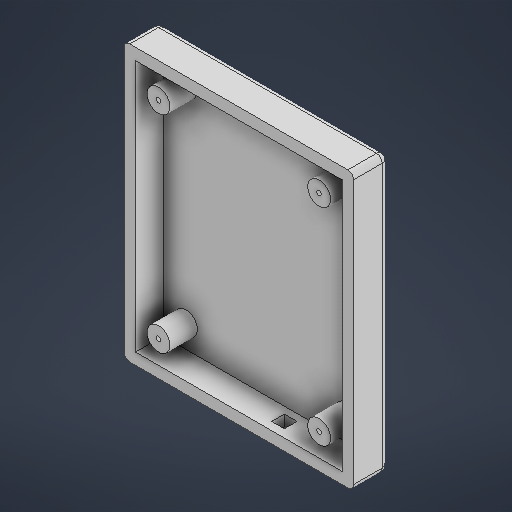
# Autodesk Inventor part: Bottom_Shell
Saved by Autodesk Inventor 2026.2 (Build 302298010, 298A)
## iProperties
Created: 2026-03-03
Part Number: Bottom_Shell
Material: Generic
Document SubType Name: Modeling
Designer: kjedr
Density: 1 g/cm^3
Appearance: Default
Author: kjedr
Autodesk Inventor part; units mm, degrees
ref_plane "YZ Plane" through (0, 0, 0) normal (1, 0, 0) x (0, 1, 0)
ref_plane "XZ Plane" through (0, 0, 0) normal (0, 1, 0) x (-1, 0, 0)
ref_plane "XY Plane" through (0, 0, 0) normal (0, 0, 1) x (1, 0, 0)
sketch "Sketch1" plane through (0, 0, 0) normal (0, 0, 1) x (1, 0, 0)
  line L0 (0, 0) -> (127, 0)
  line L1 (127, 0) -> (127, 152.4)
  line L2 (127, 152.4) -> (0, 152.4)
  line L3 (0, 152.4) -> (0, 0)
  dimension "d0" = 127
  dimension "d1" = 152.4
  constraints: 8 end point, 2 parallel, 1 horizontal, 1 perpendicular
  measures "d0" distance of L2.end L1.end
  measures "d1" distance of L1.end L0.end
extrude "Extrusion1" add sketch "Sketch1" along normal blind 19.05
sketch "Sketch2" plane through (0, 0, 19.05) normal (0, 0, 1) x (1, 0, 0)
  line L0 (6.35, 6.35) -> (120.65, 6.35)
  line L1 (120.65, 6.35) -> (120.65, 146.05)
  line L2 (120.65, 146.05) -> (6.35, 146.05)
  line L3 (6.35, 146.05) -> (6.35, 6.35)
  line L4 (0, 152.4) -> (0, 0) projected
  line L5 (0, 0) -> (127, 0) projected
  line L6 (127, 0) -> (127, 152.4) projected
  line L7 (127, 152.4) -> (0, 152.4) projected
  point P0 (127, 76.2)
  dimension "d4" = 6.35
  dimension "d5" = 6.35
  dimension "d6" = 6.35
  dimension "d7" = 6.35
  constraints: 8 end point, 2 parallel, 1 horizontal, 1 midpoint, 1 perpendicular
  measures "d4" distance between parallel lines of L4 L3
  measures "d5" distance between parallel lines of L5 L0
  measures "d6" distance from line of point (127, 76.2) L1
  measures "d7" distance between parallel lines of L7 L2
extrude "Extrusion2" cut sketch "Sketch2" against normal blind 15.24 contours L3 L2 L1 L0
fillet "Fillet1" radius 3.175 8 edges at (63.5, 152.4, 0) (127, 76.2, 0) (127, 0, 9.525) (0, 76.2, 0) (63.5, 0, 0) (127, 152.4, 9.525) (0, 152.4, 9.525) (0, 0, 9.525)
sketch "Sketch5" plane through (0, 0, 3.81) normal (0, 0, 1) x (1, 0, 0)
  circle A0 centre (19.05, 133.35) radius 6.35
  circle A1 centre (107.95, 133.35) radius 6.35
  circle A2 centre (19.05, 19.05) radius 6.35
  circle A3 centre (107.95, 19.05) radius 6.35
  line L0 (6.35, 6.35) -> (6.35, 146.05) projected
  line L1 (6.35, 146.05) -> (120.65, 146.05) projected
  line L2 (120.65, 146.05) -> (120.65, 6.35) projected
  line L3 (120.65, 6.35) -> (6.35, 6.35) projected
  point P0 (0, 0)
  dimension "d11" = 12.7
  dimension "d12" = 12.7
  dimension "d13" = 12.7
  dimension "d14" = 12.7
  dimension "d15" = 12.7
  constraints: 4 centre point, 3 equal radius, 2 horizontal alignment, 2 vertical alignment
  measures "d11" diameter of A0
  measures "d12" distance from line of L0 A0.centre
  measures "d13" distance from line of L1 A0.centre
  measures "d14" distance from line of L2 A1.centre
  measures "d15" distance from line of L3 A3.centre
extrude "Extrusion3" add sketch "Sketch5" along normal blind 15.24 contours A0 | A1 | A2 | A3
sketch "Sketch6" plane through (0, 0, 3.81) normal (0, 0, 1) x (1, 0, 0)
  line L0 (28.231, 93.35) -> (98.769, 93.35) construction
  line L1 (98.769, 93.35) -> (98.769, 9.35) construction
  line L2 (98.769, 9.35) -> (28.231, 9.35) construction
  line L3 (28.231, 9.35) -> (28.231, 93.35) construction
  circle A0 centre (32.7028, 86.056) radius 1.6
  circle A1 centre (94.3232, 86.056) radius 1.6
  circle A2 centre (32.7028, 25.35) radius 1.6
  circle A3 centre (94.3232, 25.35) radius 1.6
  line L4 (6.35, 146.05) -> (120.65, 146.05) projected
  line L5 (3.175, 0) -> (123.825, 0) projected
  line L6 (120.65, 6.35) -> (6.35, 6.35) projected
  point P0 (0, 0)
  point P1 (63.5, 93.35)
  point P2 (63.5, 146.05)
  point P3 (37.211, 36.35)
  point P4 (69.769, 21.85)
  point P5 (83.346, 9.35)
  dimension "d18" = 70.538
  dimension "d19" = 84
  dimension "d30" = 3.2
  dimension "d31" = 60.706
  dimension "d32" = 61.6204
  dimension "d33" = 16
  dimension "d34" = 4.4458
  dimension "d36" = 3
  dimension "d37" = 27
  dimension "d38" = 8.98
  dimension "d39" = 12.5
  dimension "d40" = 29
  dimension "d41" = 15.423
  constraints: 8 end point, 4 centre point, 3 equal radius, 3 vertical alignment, 2 horizontal alignment, 2 midpoint, 2 parallel, 1 horizontal, 1 perpendicular, 1 point on line
  measures "d18" distance of L1.end L2.end
  measures "d19" distance of L0.end L1.end
  measures "d30" diameter of A0
  measures "d31" distance of A2.centre A0.centre
  measures "d32" distance of A3.centre A2.centre
  measures "d33" distance from line of L2 A3.centre
  measures "d34" distance from line of L1 A3.centre
  measures "d36" distance between parallel lines of L6 L2
  measures "d37" distance from line of L2 point (37.211, 36.35)
  measures "d38" distance from line of L3 point (37.211, 36.35)
  measures "d39" distance from line of L2 point (69.769, 21.85)
  measures "d40" distance from line of L1 point (69.769, 21.85)
  measures "d41" distance from line of L1 point (83.346, 9.35)
sketch "Sketch8" plane through (0, 0, 0) normal (0, 0, -1) x (-1, 0, 0)
  circle A0 centre (-19.05, 133.35) radius 6.35 projected
  circle A1 centre (-19.05, 133.35) radius 6.35
  circle A2 centre (-107.95, 133.35) radius 6.35 projected
  circle A3 centre (-107.95, 133.35) radius 6.35
  circle A4 centre (-107.95, 19.05) radius 6.35 projected
  circle A5 centre (-107.95, 19.05) radius 6.35
  circle A6 centre (-19.05, 19.05) radius 6.35 projected
  circle A7 centre (-19.05, 19.05) radius 6.35
  point P0 (0, 0)
  constraints: 4 centre point, 4 coincident
extrude "Extrusion4" cut sketch "Sketch8" against normal blind 2.54
hole "Hole1" at (19.05, 19.05, 0) at (19.05, 133.35, 0) at (107.95, 133.35, 0) at (107.95, 19.05, 0) direction (0, 0, 1) diameter 2.54 end through all
sketch "Sketch11" plane through (3.175, 0, 3.175) normal (0, -1, 0) x (1, 0, 0)
  line L0 (123.825, 0) -> (123.825, 15.875) projected
  line L1 (74.097, 11.4375) -> (81.097, 11.4375)
  line L2 (81.097, 11.4375) -> (81.097, 4.4375)
  line L3 (81.097, 4.4375) -> (74.097, 4.4375)
  line L4 (74.097, 4.4375) -> (74.097, 11.4375)
  line L5 (74.097, 11.4375) -> (81.097, 4.4375) construction
  line L6 (81.097, 11.4375) -> (74.097, 4.4375) construction
  line L7 (120.65, 15.875) -> (120.65, 0) projected
  point P0 (-3.175, -3.175)
  point P1 (77.597, 7.9375)
  point P2 (81.097, 7.9375)
  point P3 (120.65, 7.9375)
  dimension "d42" = 46.228
  dimension "d43" = 7
  dimension "d44" = 7
  constraints: 12 end point, 4 midpoint, 2 parallel, 1 horizontal, 1 horizontal alignment, 1 perpendicular
  measures "d42" distance from line of L0 point (77.597, 7.938)
  measures "d43" distance of L2.end L3.end
  measures "d44" distance of L1.end L2.end
extrude "Extrusion5" cut sketch "Sketch11" against normal up to surface (6.35 mm away)
body "Solid1"
